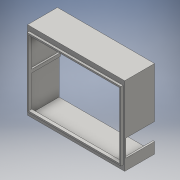
# Autodesk Inventor part: gora
Saved by Autodesk Inventor 2016 SP1 (Build 200210100, 210)
## iProperties
Created: 2019-03-01
Part Number: gora
Material: Ogólny
Document SubType Name: Modeling
Designer: Maciek
Density: 1 g/cm^3
Appearance: Domyślna
Author: Maciek
Autodesk Inventor part; units mm, degrees
ref_plane "YZ Plane" through (0, 0, 0) normal (1, 0, 0) x (0, 1, 0)
ref_plane "XZ Plane" through (0, 0, 0) normal (0, 1, 0) x (-1, 0, 0)
ref_plane "XY Plane" through (0, 0, 0) normal (0, 0, 1) x (1, 0, 0)
sketch "Szkic1" plane through (0, 0, 0) normal (0, 1, 0) x (-1, 0, 0)
  line L0 (0, 0) -> (88, 0)
  line L1 (88, 0) -> (88, 64.5)
  line L2 (88, 64.5) -> (0, 64.5)
  line L3 (0, 64.5) -> (0, 0)
  line L4 (88, 64.5) -> (86.5, 64.5) construction
  line L5 (86.5, 64.5) -> (86.5, 63) construction
  line L6 (86.5, 63) -> (88, 63) construction
  line L7 (88, 63) -> (88, 64.5) construction
  line L8 (0, 0) -> (1.5, 0) construction
  line L9 (1.5, 0) -> (1.5, 1.5) construction
  line L10 (1.5, 1.5) -> (0, 1.5) construction
  line L11 (0, 1.5) -> (0, 0) construction
  line L12 (86.5, 63) -> (1.5, 63)
  line L13 (1.5, 63) -> (1.5, 1.5)
  line L14 (1.5, 1.5) -> (86.5, 1.5)
  line L15 (86.5, 1.5) -> (86.5, 63)
  dimension "d0" = 88
  dimension "d1" = 64.5
  dimension "d2" = 1.5
  dimension "d3" = 1.5
  dimension "d4" = 1.5
  dimension "d5" = 1.5
  constraints: 32 end point, 8 parallel, 4 horizontal, 4 perpendicular
  measures "d0" distance of L2.end L1.end
  measures "d1" distance of L1.end L0.end
  measures "d2" distance of L6.end L5.end
  measures "d3" distance of L5.end L4.end
  measures "d4" distance of L10.end L9.end
  measures "d5" distance of L9.end L8.end
extrude "Wyciągnięcie proste1" add sketch "Szkic1" against normal blind 2
sketch "Szkic2" plane through (0, 0, 0) normal (0, 1, 0) x (1, 0, 0)
  line L0 (0, -64.5) -> (-88, -64.5) construction
  line L1 (0, -64.5) -> (1.5, -64.5) construction
  line L2 (1.5, -64.5) -> (1.5, -69) construction
  line L3 (1.5, -69) -> (0, -69) construction
  line L4 (0, -69) -> (0, -64.5) construction
  line L5 (-88, 0) -> (0, 0) construction
  line L6 (-88, 0) -> (-89.5, 0) construction
  line L7 (-89.5, 0) -> (-89.5, 4.5) construction
  line L8 (-89.5, 4.5) -> (-88, 4.5) construction
  line L9 (-88, 4.5) -> (-88, 0) construction
  line L10 (1.5, -69) -> (-89.5, -69)
  line L11 (-89.5, -69) -> (-89.5, 4.5)
  line L12 (-89.5, 4.5) -> (1.5, 4.5)
  line L13 (1.5, 4.5) -> (1.5, -69)
  line L14 (-86.5, -1.5) -> (-86.5, -63) projected
  line L15 (-1.5, -63) -> (-86.5, -63)
  line L16 (-86.5, -63) -> (-86.5, -1.5)
  line L17 (-86.5, -1.5) -> (-1.5, -1.5)
  line L18 (-1.5, -1.5) -> (-1.5, -63)
  dimension "d8" = 1.5
  dimension "d9" = 4.5
  dimension "d10" = 1.5
  dimension "d11" = 4.5
  constraints: 32 end point, 8 parallel, 4 horizontal, 4 perpendicular
  measures "d8" distance of L2.end L3.end
  measures "d9" distance of L1.end L2.end
  measures "d10" distance of L7.end L8.end
  measures "d11" distance of L6.end L7.end
extrude "Wyciągnięcie proste2" add sketch "Szkic2" along normal blind 1
sketch "Szkic3" plane through (0, 1, 0) normal (0, 1, 0) x (1, 0, 0)
  line L0 (-89.5, -69) -> (1.5, -69) construction
  line L1 (1.5, -69) -> (0, -69) construction
  line L2 (0, -69) -> (0, -67.5) construction
  line L3 (0, -67.5) -> (1.5, -67.5) construction
  line L4 (1.5, -67.5) -> (1.5, -69) construction
  line L5 (-89.5, 4.5) -> (-89.5, -69) construction
  line L6 (-89.5, 4.5) -> (-88, 4.5) construction
  line L7 (-88, 4.5) -> (-88, 3) construction
  line L8 (-88, 3) -> (-89.5, 3) construction
  line L9 (-89.5, 3) -> (-89.5, 4.5) construction
  line L10 (0, -67.5) -> (-88, -67.5)
  line L11 (-88, -67.5) -> (-88, 3)
  line L12 (-88, 3) -> (0, 3)
  line L13 (0, 3) -> (0, -67.5)
  line L14 (1.5, 4.5) -> (-89.5, 4.5) projected
  line L15 (1.5, -69) -> (-89.5, -69)
  line L16 (-89.5, -69) -> (-89.5, 4.5)
  line L17 (-89.5, 4.5) -> (1.5, 4.5)
  line L18 (1.5, 4.5) -> (1.5, -69)
  point P0 (0, 0)
  dimension "d14" = 1.5
  dimension "d15" = 1.5
  dimension "d16" = 1.5
  dimension "d17" = 1.5
  constraints: 32 end point, 8 parallel, 4 horizontal, 4 perpendicular
  measures "d14" distance of L2.end L3.end
  measures "d15" distance of L1.end L2.end
  measures "d16" distance of L7.end L8.end
  measures "d17" distance of L6.end L7.end
extrude "Wyciągnięcie proste3" add sketch "Szkic3" along normal blind 27
sketch "Szkic4" plane through (0, 1, -3) normal (-1, 0, 0) x (0, 0, 1)
  line L0 (72, -1) -> (67.5, -1) projected
  line L1 (67.5, -1) -> (3, -1) projected
  line L2 (3, -1) -> (-1.5, -1) projected
  line L3 (-1.5, -1) -> (-1.5, 27) projected
  line L4 (-1.5, 27) -> (0, 27) projected
  line L5 (0, 27) -> (70.5, 27) projected
  line L6 (70.5, 27) -> (72, 27) projected
  line L7 (72, 27) -> (72, -1) projected
  line L8 (67.5, -1) -> (67.5, -3) projected
  line L9 (67.5, -3) -> (3, -3) projected
  line L10 (3, -3) -> (3, -1) projected
  line L11 (0, 27) -> (0, 0) projected
  line L12 (0, 0) -> (70.5, 0) projected
  line L13 (70.5, 0) -> (70.5, 27) projected
  line L14 (72, -1) -> (67.5, -1) projected
  line L15 (67.5, -1) -> (3, -1) projected
  line L16 (3, -1) -> (-1.5, -1) projected
  line L17 (-1.5, -1) -> (-1.5, 27) projected
  line L18 (-1.5, 27) -> (0, 27) projected
  line L19 (0, 27) -> (70.5, 27) projected
  line L20 (70.5, 27) -> (72, 27) projected
  line L21 (72, 27) -> (72, -1) projected
  line L22 (67.5, -1) -> (67.5, -3) projected
  line L23 (67.5, -3) -> (3, -3) projected
  line L24 (3, -3) -> (3, -1) projected
  line L25 (0, 27) -> (0, 0) projected
  line L26 (0, 0) -> (70.5, 0) projected
  line L27 (70.5, 0) -> (70.5, 27) projected
  line L28 (0, 0) -> (8.65, 0) construction
  line L29 (70.5, 0) -> (0, 0) construction
  line L30 (8.65, 0) -> (24.95, 0) construction
  line L31 (8.65, 0) -> (24.95, 0)
  line L32 (24.95, 0) -> (24.95, 27)
  line L33 (24.95, 27) -> (8.65, 27)
  line L34 (8.65, 27) -> (8.65, 0)
  dimension "d20" = 8.65
  dimension "d21" = 16.3
  constraints: 12 end point, 3 point on line, 2 parallel, 1 horizontal, 1 perpendicular
  measures "d20" distance of L11.end L28.end
  measures "d21" distance of L28.end L30.end
extrude "Wyciągnięcie proste4" cut sketch "Szkic4" against normal blind 1.5 contours L32 L12 L34 L5
sketch "Szkic5" plane through (0, 1, 0) normal (0, 1, 0) x (1, 0, 0)
  line L0 (-88, 3) -> (-88, -67.5) construction
  line L1 (-88, 3) -> (-88, -30.9) construction
  line L2 (-88, -30.9) -> (-86.5, -30.9)
  line L3 (-86.5, -30.9) -> (-86.5, -33.9)
  line L4 (-86.5, -33.9) -> (-88, -33.9)
  line L5 (-88, -33.9) -> (-88, -30.9)
  point P0 (0, 0)
  dimension "d24" = 33.9
  dimension "d25" = 1.5
  dimension "d26" = 3
  constraints: 10 end point, 2 parallel, 1 horizontal, 1 perpendicular, 1 point on line
  measures "d24" distance of L0.start L1.end
  measures "d25" distance of L3.end L4.end
  measures "d26" distance of L2.end L3.end
extrude "Wyciągnięcie proste5" add sketch "Szkic5" along normal blind 27
sketch "Szkic6" plane through (0, 1, 0) normal (0, 1, 0) x (1, 0, 0)
  line L0 (-1.5, -1.5) -> (-1.5, -63) construction
  line L1 (-1.5, -63) -> (-1.5, -26) construction
  line L2 (-1.5, -63) -> (-16.5, -63) construction
  line L3 (-1.5, -63) -> (-86.5, -63) construction
  line L4 (-1.5, -26) -> (-1.5, -63)
  line L5 (-16.5, -63) -> (-1.5, -63)
  line L6 (-16.5, -63) -> (-16.5, -67.5)
  line L7 (0, -67.5) -> (-88, -67.5) projected
  line L8 (-16.5, -67.5) -> (0, -67.5)
  line L9 (0, -67.5) -> (0, -26)
  line L10 (0, -21.95) -> (0, -67.5) projected
  line L11 (-1.5, -26) -> (0, -26)
  point P0 (0, 0)
  dimension "d29" = 37
  dimension "d30" = 15
  constraints: 16 end point, 4 point on line, 2 collinear, 2 perpendicular, 1 vertical
  measures "d29" distance of L0.end L1.end
  measures "d30" distance of L0.end L2.end
extrude "Wyciągnięcie proste6" add sketch "Szkic6" along normal blind 25
